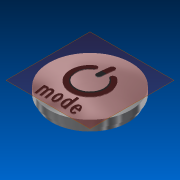
# Autodesk Inventor part: GoPro Hero 3 Mode Button
Saved by Autodesk Inventor 2015 (Build 190159000, 159)
## iProperties
Created: 2013-02-15
Material: ABS Plastic
Document SubType Name: Modeling
Designer: sdarley
Density: 1 g/cm^3
Project: GoPro Hero 3 HD Camera
Description: GoPro Hero 3 Mode Button
Appearance: Silver
Author: sdarley
Title: GoPro Hero 3 Mode Button
Revision Number: 1
Autodesk Inventor part; units mm, degrees
note: some values were not read from the file. Chosen so that the rebuilt part matches the saved one: direction of "Emboss1".
ref_plane "YZ Plane" through (0, 0, 0) normal (1, 0, 0) x (0, 1, 0)
ref_plane "XZ Plane" through (0, 0, 0) normal (0, 1, 0) x (-1, 0, 0)
ref_plane "XY Plane" through (0, 0, 0) normal (0, 0, 1) x (1, 0, 0)
sketch "Sketch1" plane through (0, 0, 0) normal (0, 1, 0) x (-1, 0, 0)
  line L0 (5.5, -0.75) -> (5.5, 0)
  line L1 (5.5, 0) -> (5.9, 0)
  line L2 (5.9, 0) -> (5.9, 1)
  line L3 (5.5, -0.75) -> (0, -0.75)
  line L4 (0, -0.75) -> (0, 1.75)
  arc A0 (5.9, 1) -> (0, 1.75) centre (0, -21.8317) ccw
  point P0 (0, 0)
  point P1 (0, 0)
  dimension "d0" = 5.5
  dimension "d2" = 5.9
  dimension "d3" = 0.75
  dimension "d4" = 1.75
  dimension "d5" = 2.5
  constraints: 10 end point, 3 perpendicular, 2 point on circle, 1 centre point, 1 coincident, 1 horizontal, 1 horizontal alignment, 1 line through centre, 1 parallel, 1 vertical alignment
  measures "d0" distance between parallel lines of L4 L0
  measures "d2" distance between parallel lines of L4 L2
  measures "d3" distance between parallel lines of L3 L1
  measures "d4" distance from line of L2.end L3
  measures "d5" distance of L3.end L4.end
revolve "Revolution1" add sketch "Sketch1" angle 360 about axis through (0, 0, -0.75) along (0, 0, 1)
ref_plane "Work Plane1" through (0, 0, 1.75) normal (0, 0, -1) x (-1, 0, 0)
sketch "Sketch2" plane through (0, 0, 1.75) normal (0, 0, -1) x (-1, 0, 0)
  arc A0 (-1.125, 1.6536) -> (1.125, 1.6536) centre (0, 0) ccw
  arc A1 (-1.575, 2.315) -> (1.575, 2.315) centre (0, 0) ccw
  line L0 (-0.35, 3.25) -> (-0.35, 1.25)
  line L1 (0.35, 1.25) -> (0.35, 3.25)
  arc A2 (1.575, 2.315) -> (1.125, 1.6536) centre (1.35, 1.9843) ccw
  arc A3 (-1.125, 1.6536) -> (-1.575, 2.315) centre (-1.35, 1.9843) ccw
  arc A4 (-0.35, 1.25) -> (0.35, 1.25) centre (0, 1.25) ccw
  arc A5 (0.35, 3.25) -> (-0.35, 3.25) centre (0, 3.25) ccw
  line L2 (0.35, 0.9) -> (-0.35, 0.9) construction
  line L3 (3.1, -2.9) -> (-3.1, -2.9) construction
  line L4 (3.1, -4.9) -> (-3.1, -4.9) construction
  line L5 (3.1, -2.9) -> (3.1, -4.9) construction
  line L6 (-3.1, -2.9) -> (-3.1, -4.9) construction
  ellipse E0 centre (-0.8196, -4.2) end of major axis (-0.8196, -4.73) minor radius 0.2
  ellipse E1 centre (-0.8196, -4.2) end of major axis (-0.8196, -4.9) minor radius 0.5 (-1.0196, -4.8416) -> (-1.0196, -3.5584) ccw
  line L7 (-1.3196, -4.9) -> (-1.0196, -4.9)
  line L8 (-1.0196, -2.9) -> (-1.3196, -2.9)
  line L9 (-1.3196, -2.9) -> (-1.3196, -4.9)
  line L10 (3.1, -3.5) -> (-3.1, -3.5) construction
  line L11 (-1.0196, -4.9) -> (-1.0196, -4.8416)
  line L12 (-1.0196, -3.5584) -> (-1.0196, -2.9)
  ellipse E2 centre (0.4991, -4.2) end of major axis (0.4991, -3.5) minor radius 0.5
  ellipse E3 centre (0.4991, -4.2) end of major axis (0.4991, -3.7128) minor radius 0.2
  line L13 (3.0993, -3.5) -> (3.0993, -4.9)
  line L14 (3.0993, -4.9) -> (2.7993, -4.9)
  line L15 (2.7993, -3.9716) -> (2.7993, -4.9)
  line L16 (3.0993, -3.5) -> (2.7993, -3.5)
  line L17 (2.7993, -3.5) -> (2.7993, -3.5323)
  line L18 (2.3835, -3.9716) -> (2.3835, -4.9)
  line L19 (2.0835, -3.9716) -> (2.0835, -4.9)
  line L20 (1.6677, -3.9716) -> (1.6677, -4.9)
  line L21 (1.3677, -3.9716) -> (1.3677, -4.9)
  line L22 (1.6677, -4.9) -> (1.3677, -4.9)
  line L23 (2.3835, -4.9) -> (2.0835, -4.9)
  arc A6 (2.7993, -3.9716) -> (2.3835, -3.9716) centre (2.5914, -3.9716) ccw
  arc A7 (2.0835, -3.9716) -> (1.6677, -3.9716) centre (1.8756, -3.9716) ccw
  arc A8 (2.2335, -3.7128) -> (1.3677, -3.9716) centre (1.8392, -3.9716) ccw
  arc A9 (2.7993, -3.5323) -> (2.2335, -3.7128) centre (2.6277, -3.9716) ccw
  ellipse E4 centre (-2.1719, -4.2) end of major axis (-2.1719, -3.5) minor radius 0.5 (-2.6012, -4.5589) -> (-2.6719, -4.2004) ccw
  line L24 (-1.9719, -4.1999) -> (-2.6719, -4.2004)
  line L25 (-1.9823, -4.0314) -> (-2.3615, -4.0317)
  ellipse E5 centre (-2.1719, -4.2) end of major axis (-2.1719, -3.67) minor radius 0.2 (-1.9823, -4.0314) -> (-2.3615, -4.0317) ccw
  ellipse E6 centre (-2.1719, -4.2) end of major axis (-2.1719, -3.67) minor radius 0.2 (-2.3385, -4.4934) -> (-1.9719, -4.1999) ccw
  line L26 (-2.3385, -4.4934) -> (-2.6012, -4.5589)
  line L27 (-2.2311, -3.67) -> (-2.7669, -3.67) construction
  line L28 (-0.5722, -3.67) -> (-1.0196, -3.67) construction
  line L29 (-2.006, -4.73) -> (-2.3328, -4.73) construction
  point P0 (0, 0.9)
  point P1 (0, -2.8)
  point P2 (0, -2.9)
  point P3 (2.2335, -4.9)
  dimension "d22" = 0.5
  dimension "d23" = 0.5
  dimension "d24" = 0.2
  dimension "d29" = 0.5
  dimension "d31" = 0.2
  dimension "d32" = 0.2
  dimension "d8" = 2
  dimension "d10" = 2.8
  dimension "d11" = 0.7
  dimension "d12" = 2.7
  dimension "d13" = 0.9
  dimension "d14" = 1.9
  dimension "d17" = 2
  dimension "d18" = 0.1
  dimension "d19" = 6.2
  dimension "d20" = 1.4
  dimension "d21" = 0.3
  dimension "d25" = 0.3
  dimension "d26" = 0.3
  dimension "d27" = 0.3
  dimension "d28" = 0.3
  dimension "d33" = 0.17
  dimension "d34" = 0.17
  dimension "d35" = 0.17
  constraints: 58 end point, 22 point on circle, 14 tangent, 13 horizontal, 12 vertical, 10 centre point, 9 parallel, 7 perpendicular, 5 coincident, 5 point on line, 4 vertical alignment, 3 equal radius, 3 horizontal alignment, 3 midpoint, 1 collinear, 32 other
  measures "d8" radius of A0
  measures "d10" radius of A1
  measures "d11" distance between parallel lines of L0 L1
  measures "d13" distance from line of L2 point (0, 0)
  measures "d18" distance edge to line of A1 L3
  measures "d19" distance between parallel lines of L6 L5
  measures "d21" distance between parallel lines of L9 L12
  measures "d25" distance between parallel lines of L15 L13
  measures "d26" distance between parallel lines of L19 L18
  measures "d27" distance between parallel lines of L21 L20
  measures "d33" distance between parallel lines of L10 L27
  measures "d34" distance between parallel lines of L10 L28
emboss "Emboss1" sketch "Sketch2" operation add depth 0.1 direction (0, 0, -1)
equation "\"d23\" = d22"
equation "\"d24\" = d23 - d21"
equation "\"d29\" = d22"
equation "\"d25\" = d21"
equation "\"d26\" = d25"
equation "\"d27\" = d25"
equation "\"d28\" = d25"
body "Solid1"
